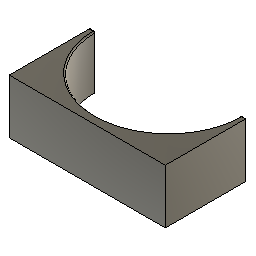
wheel_stop (Autodesk Fusion 360 design; units mm, degrees)
Autodesk Fusion 360 part; units mm, degrees
sketch "Sketch1" plane through (0, 0, 0) normal (0, 0, 1) x (1, 0, 0)
  line L0 (0, 0) -> (-230, 0)
  line L1 (-230, 0) -> (-230, 120)
  line L2 (-230, 120) -> (0, 120)
  line L3 (0, 120) -> (0, 0)
  dimension "d1" = 120
  dimension "d2" = 230
  constraint horizontal L0
  constraint vertical L1
  constraint horizontal L2
  constraint vertical L3
  constraint coincident L0.start L3.end
  measures "d1" distance of L0.start L2.end
  measures "d2" distance of L0.start L0.end
extrude "Extrude1" add sketch "Sketch1" along normal blind 80
sketch "Sketch2" plane through (0, 0, 80) normal (0, 0, 1) x (-1, 0, 0)
  line L0 (0, -120) -> (230, -120)
  line L1 (230, -120) -> (230, 0)
  line L2 (230, 0) -> (0, 0)
  line L3 (0, 0) -> (0, -120)
  circle A0 centre (115, -120) radius 107.5
  dimension "d5" = 215
  constraint midpoint L0 A0.centre
  measures "d5" diameter of A0
extrude "Extrude2" cut sketch "Sketch2" against normal blind 170 contours L0 A0 picked at (128.0914, -86.6437)
fillet "Fillet1" radius 2 10 edges at (-222.5, 120, 40) (-230, 120, 40) (-7.5, 120, 40) (0, 120, 40) (-115, 12.5, 80) (-115, 12.5, 0) (-3.75, 120, 80) (-3.75, 120, 0) (-226.25, 120, 80) (-226.25, 120, 0)
